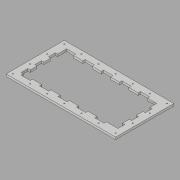
# Autodesk Inventor part: b_Base_support 1
Saved by Autodesk Inventor 2019 (Build 230136000, 136)
## iProperties
Created: 2021-11-07
Part Number: b_Base_support 1
Material: Generic
Document SubType Name: Modeling
Designer: Mohamed
Density: 1 g/cm^3
Appearance: Default
Author: Mohamed
Autodesk Inventor part; units mm, degrees
ref_plane "YZ Plane" through (0, 0, 0) normal (1, 0, 0) x (0, 1, 0)
ref_plane "XZ Plane" through (0, 0, 0) normal (0, 1, 0) x (-1, 0, 0)
ref_plane "XY Plane" through (0, 0, 0) normal (0, 0, 1) x (1, 0, 0)
sketch "Sketch1" plane through (0, 0, 0) normal (0, 1, 0) x (-1, 0, 0)
  line L0 (0, 0) -> (320, 0)
  line L1 (320, 0) -> (320, -170)
  line L2 (320, -170) -> (0, -170)
  line L3 (0, -170) -> (0, 0)
  line L4 (0, 0) -> (25, 0)
  line L5 (25, -25) -> (295, -25)
  line L6 (295, -25) -> (295, -145)
  line L7 (295, -145) -> (25, -145)
  line L8 (25, -145) -> (25, -25)
  dimension "d0" = 320
  dimension "d1" = 170
  dimension "d2" = 25
  dimension "d3" = 25
  dimension "d4" = 270
  dimension "d5" = 120
  constraints: 18 end point, 5 perpendicular, 2 parallel, 1 horizontal, 1 point on line
  measures "d0" distance of L1.end L2.end
  measures "d1" distance of L0.end L1.end
  measures "d2" distance of L0.start L4.end
  measures "d3" distance of L4.end L5.start
  measures "d4" distance of L5.start L5.end
  measures "d5" distance of L5.end L6.end
extrude "Extrusion1" add sketch "Sketch1" along normal blind 6.7
sketch "Sketch2" plane through (0, 6.7, 0) normal (0, 1, 0) x (1, 0, 0)
  line L0 (-320, 0) -> (0, 0) projected
  line L1 (0, 0) -> (0, 170) projected
  circle A0 centre (-10, 10) radius 1.6
  line L2 (0, 170) -> (0, 160)
  circle A1 centre (-10, 160) radius 1.6
  dimension "d10" = 3.2
  dimension "d13" = 3.2
  constraints: 2 centre point, 2 end point, 1 point on line
  measures "d10" diameter of A0
  measures "d13" diameter of A1
extrude "Extrusion2" cut sketch "Sketch2" against normal blind 6.7
pattern_linear "Rectangular Pattern1" count 7 spacing 50 along (-1, 0, 0) of "Extrusion2"
sketch "Sketch3" plane through (0, 6.7, 0) normal (0, 1, 0) x (1, 0, 0)
  circle A0 centre (-310, 10) radius 1.6 projected
  circle A1 centre (-310, 60) radius 1.6
  circle A2 centre (-10, 10) radius 1.6 projected
  circle A3 centre (-10, 60) radius 1.6
  point P0 (0, 0)
  dimension "d20" = 3.2
  dimension "d22" = 3.2
  constraints: 2 centre point
  measures "d20" diameter of A1
  measures "d22" diameter of A3
extrude "Extrusion3" cut sketch "Sketch3" against normal blind 6.7 contours A1 | A3
pattern_linear "Rectangular Pattern2" count 2 spacing 50 along (0, 0, -1) of "Extrusion3"
sketch "Sketch4" plane through (0, 6.7, 0) normal (0, 1, 0) x (1, 0, 0)
  line L0 (-25, 25) -> (-25, 145) projected
  line L1 (-25, 25) -> (-295, 25) projected
  line L2 (-52, 25) -> (-79, 25)
  line L3 (-79, 25) -> (-79, 18.3)
  line L4 (-79, 18.3) -> (-52, 18.3)
  line L5 (-52, 18.3) -> (-52, 25)
  line L6 (-295, 145) -> (-25, 145) projected
  line L7 (-25, 145) -> (-52, 145)
  line L8 (-52, 145) -> (-79, 145)
  line L9 (-79, 145) -> (-79, 151.7)
  line L10 (-79, 151.7) -> (-52, 151.7)
  line L11 (-52, 151.7) -> (-52, 145)
  point P0 (0, 0)
  dimension "d28" = 27
  dimension "d29" = 27
  dimension "d30" = 6.7
  dimension "d31" = 27
  dimension "d32" = 27
  dimension "d33" = 6.7
  constraints: 18 end point, 4 parallel, 2 horizontal, 2 perpendicular, 2 point on line
  measures "d28" distance of L0.start L2.start
  measures "d29" distance of L4.end L3.end
  measures "d30" distance of L3.end L2.end
  measures "d31" distance of L0.end L7.end
  measures "d32" distance of L9.end L10.end
  measures "d33" distance of L8.end L9.end
extrude "Extrusion4" cut sketch "Sketch4" against normal blind 6.7
pattern_linear "Rectangular Pattern3" count 5 spacing 54 along (-1, 0, 0) of "Extrusion4"
sketch "Sketch5" plane through (0, 6.7, 0) normal (0, 1, 0) x (1, 0, 0)
  line L0 (-25, 145) -> (-25, 25) projected
  line L1 (-25, 25) -> (-18.3, 25)
  line L2 (-18.3, 25) -> (-18.3, 45)
  line L3 (-18.3, 45) -> (-25, 45)
  line L4 (-25, 45) -> (-25, 25)
  line L5 (-295, 18.3) -> (-295, 151.7) projected
  line L6 (-295, 25) -> (-301.7, 25)
  line L7 (-301.7, 25) -> (-301.7, 45)
  line L8 (-301.7, 45) -> (-295, 45)
  line L9 (-295, 45) -> (-295, 25)
  point P0 (0, 0)
  dimension "d39" = 6.7
  dimension "d40" = 20
  dimension "d41" = 6.7
  dimension "d42" = 20
  constraints: 16 end point, 4 parallel, 2 horizontal, 2 perpendicular, 1 point on line
  measures "d39" distance of L3.end L2.end
  measures "d40" distance of L2.end L1.end
  measures "d41" distance of L7.end L8.end
  measures "d42" distance of L6.end L7.end
extrude "Extrusion5" cut sketch "Sketch5" against normal blind 6.7
pattern_linear "Rectangular Pattern4" count 3 spacing 40 along (0, 0, -1) of "Extrusion5"
body "Solid1"
